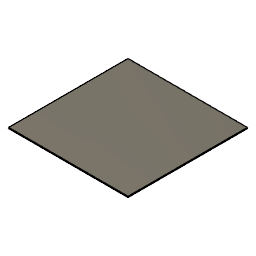
shim (Autodesk Fusion 360 design; units mm, degrees)
part number: 2026-08-14-18-01-15-515
Autodesk Fusion 360 part; units mm, degrees
sketch "Sketch1" plane through (0, 0, 0) normal (0, 1, 0) x (1, 0, 0)
  line L0 (-12.855, 9.4832) -> (107.145, 9.4832)
  line L1 (107.145, 9.4832) -> (107.145, -110.5168)
  line L2 (107.145, -110.5168) -> (-12.855, -110.5168)
  line L3 (-12.855, -110.5168) -> (-12.855, 9.4832)
  dimension "d1" = 120
  dimension "d2" = 120
  constraint horizontal L0
  constraint vertical L1
  constraint horizontal L2
  constraint vertical L3
  measures "d1" distance of L0.start L0.end
  measures "d2" distance of L0.start L2.end
extrude "Extrude1" add sketch "Sketch1" along normal blind 0.5 makes body 1
extrude "Extrude2" add 1 faces at (27.145, 0.5, 30.5168) along direction (0, 1, 0) blind 0.5 separate body on bodies 1 makes body 2
